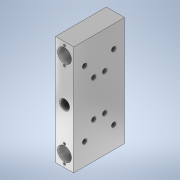
# Autodesk Inventor part: Bloque - Vinculo Cabezal
Saved by Autodesk Inventor 2020 (Build 240168000, 168)
## iProperties
Created: 2020-05-17
Part Number: Bloque - Vinculo Cabezal
Material: Aluminum 6061
Document SubType Name: Modeling
Designer: Dante
Density: 2.7 g/cm^3
Appearance: Aluminum - Dark
Mass: 559.283 g
Surface Area: 455.426 cm^2
Volume: 207.142 cm^3
Author: Dante
Autodesk Inventor part; units mm, degrees
ref_plane "YZ Plane" through (0, 0, 0) normal (1, 0, 0) x (0, 1, 0)
ref_plane "XZ Plane" through (0, 0, 0) normal (0, 1, 0) x (-1, 0, 0)
ref_plane "XY Plane" through (0, 0, 0) normal (0, 0, 1) x (1, 0, 0)
sketch "Sketch1" plane through (0, 0, 0) normal (0, 0, 1) x (1, 0, 0)
  line L0 (14.1854, 26.7901) -> (14.1854, -123.2099)
  line L1 (14.1854, -123.2099) -> (39.1854, -123.2099)
  line L2 (39.1854, -123.2099) -> (39.1854, 26.7901)
  line L3 (39.1854, 26.7901) -> (14.1854, 26.7901)
  circle A0 centre (26.6854, 10.2901) radius 9.5
  circle A1 centre (26.6854, -48.2099) radius 6
  circle A2 centre (37.1854, -8.2099) radius 3
  line L4 (39.1854, -5.2099) -> (14.1854, -5.2099)
  line L5 (39.1854, -11.2099) -> (14.1854, -11.2099)
  circle A3 centre (26.6854, 23.2901) radius 1.5
  line L6 (26.6854, 19.7901) -> (20.6854, 19.7901)
  line L7 (26.6854, 21.7901) -> (21.9472, 21.7901)
  line L8 (26.6854, 24.7901) -> (23.6854, 24.7901)
  line L9 (26.6854, 10.2901) -> (21.9472, 10.2901)
  circle A4 centre (26.6854, -2.7099) radius 1.5
  line L10 (14.1854, -48.2099) -> (17.1854, -48.2099)
  circle A5 centre (26.6854, -106.7099) radius 9.5
  circle A6 centre (37.1854, -88.2099) radius 3
  line L11 (39.1854, -91.2099) -> (14.1854, -91.2099)
  line L12 (39.1854, -85.2099) -> (14.1854, -85.2099)
  circle A7 centre (26.6854, -119.7099) radius 1.5
  line L13 (26.6854, -116.2099) -> (20.6854, -116.2099)
  line L14 (26.6854, -118.2099) -> (21.9472, -118.2099)
  line L15 (26.6854, -121.2099) -> (23.6854, -121.2099)
  line L16 (26.6854, -106.7099) -> (21.9472, -106.7099)
  circle A8 centre (26.6854, -93.7099) radius 1.5
  dimension "d0" = 150
  dimension "d1" = 25
  dimension "d6" = 12.5
  dimension "d8" = 12
  dimension "d12" = 75
  dimension "d13" = 6
  dimension "d33" = 3
  dimension "d81" = 3.5
  dimension "d83" = 2
  dimension "d84" = 2
  dimension "d85" = 16.5
  dimension "d130" = 12.5
  dimension "d131" = 12.5
  constraints: 34 end point, 16 symmetric about line, 8 horizontal, 7 centre point, 4 point on circle, 4 point on line, 3 perpendicular, 2 vertical alignment, 1 midpoint, 1 parallel, 1 tangent, 1 vertical, 8 other
  measures "d0" distance of L0.start L0.end
  measures "d1" distance of L0.end L1.end
  measures "d6" distance from line of L9.start L2
  measures "d8" diameter of A1
  measures "d12" distance from line of L3 A1.centre
  measures "d13" diameter of A2
  measures "d33" diameter of A3
  measures "d81" distance from line of L3 A3.centre
  measures "d83" distance between parallel lines of L3 L8
  measures "d84" distance between parallel lines of L6 L7
  measures "d85" distance from line of L3 L9.start
  measures "d130" distance from line of A1.centre L2
  measures "d131" distance from line of L16.start L2
extrude "Extrusion1" add sketch "Sketch1" along normal blind 70 contours L3 L2 L4 L0 | L4 A2 L5 L0 | L5 L2 L12 L0 | L4 L2 A2 | A2 L2 | A2 L2 L5 | L12 A6 L11 L0 | L11 L2 L1 L0 | L12 L2 A6 | A6 L2 | A6 L2 L11 | A3 | A4 | A7 | A8 picked at (35.982, -7.4645) picked at (36.2539, -87.8584)
sketch "Sketch2" plane through (39.1854, -123.2099, 0) normal (1, 0, 0) x (0, 0, -1)
  circle A0 centre (-27.5, 100) radius 3
  circle A1 centre (-42.5, 100) radius 3
  circle A2 centre (-55, 120) radius 3
  circle A3 centre (-15, 120) radius 3
  line L0 (0, 150) -> (-70, 150) projected
  line L1 (0, 0) -> (0, 150) projected
  line L2 (-70, 0) -> (-70, 150) projected
  line L3 (0, 75) -> (-12, 75)
  circle A4 centre (-27.5, 50) radius 3
  circle A5 centre (-42.5, 50) radius 3
  circle A6 centre (-55, 30) radius 3
  circle A7 centre (-15, 30) radius 3
  dimension "d17" = 6
  dimension "d18" = 6
  dimension "d19" = 6
  dimension "d20" = 6
  dimension "d21" = 30
  dimension "d24" = 30
  dimension "d25" = 15
  dimension "d26" = 15
  dimension "d204" = 50
  dimension "d205" = 50
  dimension "d206" = 12.5
  dimension "d207" = 12.5
  constraints: 8 centre point, 4 symmetric about line, 2 end point, 1 horizontal, 1 midpoint, 4 other
  measures "d17" diameter of A0
  measures "d18" diameter of A1
  measures "d19" diameter of A2
  measures "d20" diameter of A3
  measures "d21" distance from line of L0 A3.centre
  measures "d24" distance from line of L0 A2.centre
  measures "d25" distance from line of A3.centre L1
  measures "d26" distance from line of L2 A2.centre
  measures "d204" distance from line of L0 A1.centre
  measures "d205" distance from line of L0 A0.centre
  measures "d206" horizontal distance of A2.centre A1.centre
  measures "d207" horizontal distance of A3.centre A0.centre
sketch "Sketch5" plane through (0, 0, 0) normal (0, 0, -1) x (-1, 0, 0)
  circle A0 centre (-26.6854, 22.2901) radius 1.5
  line L0 (-39.1854, 26.7901) -> (-14.1854, 26.7901) projected
  circle A1 centre (-26.6854, 10.2901) radius 9.5 projected
  line L1 (-14.1854, 26.7901) -> (-14.1854, -123.2099) projected
  circle A2 centre (-26.6854, -1.7099) radius 1.5
  line L2 (-14.1854, 26.7901) -> (-14.1854, -123.2099) projected
  line L3 (-14.1854, -48.2099) -> (-19.6815, -48.2099)
  circle A3 centre (-26.6854, -118.7099) radius 1.5
  circle A4 centre (-26.6854, -94.7099) radius 1.5
  circle A5 centre (-26.6854, 10.2901) radius 9.5 projected
  line L4 (-26.6854, 0.7901) -> (-19.8619, 0.7901)
  dimension "d53" = 3
  dimension "d55" = 12.5
  dimension "d56" = 3
  dimension "d58" = 12.5
  dimension "d79" = 12
  dimension "d199" = 12
  constraints: 4 centre point, 4 end point, 3 horizontal, 2 symmetric about line, 1 midpoint, 1 vertical alignment, 3 other
  measures "d53" diameter of A0
  measures "d55" distance from line of A0.centre L1
  measures "d56" diameter of A2
  measures "d58" distance from line of A2.centre L1
  measures "d79" distance of A2.centre A1.centre
  measures "d199" distance of A1.centre A0.centre
sketch "Sketch7" plane through (0, 0, 70) normal (0, 0, 1) x (1, 0, 0)
  circle A0 centre (26.6854, 22.2901) radius 1.5
  line L0 (39.1854, 26.7901) -> (14.1854, 26.7901) projected
  line L1 (39.1854, -123.2099) -> (39.1854, 26.7901) projected
  circle A1 centre (26.6854, -1.7099) radius 1.5
  line L2 (39.1854, -48.2099) -> (34.5459, -48.2099)
  circle A2 centre (26.6854, -118.7099) radius 1.5
  line L3 (39.1854, -123.2099) -> (14.1854, -123.2099)
  line L4 (39.1854, 26.7901) -> (39.1854, -123.2099)
  line L5 (26.6854, -106.7099) -> (25.3096, -106.7099)
  circle A3 centre (26.6854, -94.7099) radius 1.5
  circle A4 centre (26.6854, 10.2901) radius 9.5 projected
  dimension "d87" = 3
  dimension "d89" = 12.5
  constraints: 8 end point, 5 symmetric about line, 4 centre point, 1 horizontal, 1 midpoint, 2 other
  measures "d87" diameter of A0
  measures "d89" distance from line of L1 A0.centre
thread "Thread16" size "M12x1.5" class "6H" standard "ISO Metric profile" length 40
sketch "Sketch8" plane through (0, 0, 0) normal (0, 0, -1) x (-1, 0, 0)
  line L0 (-39.1854, -48.2099) -> (-26.6854, -48.2099)
  circle A0 centre (-26.6854, -48.2099) radius 11
  circle A1 centre (-26.6854, -48.2099) radius 6 projected
  point P0 (0, 0)
  dimension "d113" = 12.5
  dimension "d114" = 22
  constraints: 2 end point, 1 centre point, 1 coincident, 1 concentric, 1 horizontal
  measures "d113" distance of L0.start L0.end
  measures "d114" diameter of A0
extrude "Extrusion9" cut sketch "Sketch8" against normal blind 10
sketch "Sketch9" plane through (0, 0, 0) normal (0, 0, -1) x (-1, 0, 0)
  circle A0 centre (-26.6854, -48.2099) radius 11
  circle A1 centre (-26.6854, -48.2099) radius 11 projected
  circle A2 centre (-26.6854, -34.2099) radius 1.5
  circle A3 centre (-26.6854, -62.2099) radius 1.5
  line L0 (-39.1854, -123.2099) -> (-39.1854, 26.7901) projected
  line L1 (-14.1854, 26.7901) -> (-14.1854, -123.2099) projected
  dimension "d117" = 22
  dimension "d118" = 3
  dimension "d119" = 3
  dimension "d120" = 14
  dimension "d121" = 14
  dimension "d122" = 12.5
  dimension "d123" = 12.5
  constraints: 3 centre point, 1 concentric
  measures "d117" diameter of A0
  measures "d118" diameter of A2
  measures "d119" diameter of A3
  measures "d120" distance of A2.centre A0.centre
  measures "d121" distance of A0.centre A3.centre
  measures "d122" distance from line of L0 A2.centre
  measures "d123" distance from line of L1 A3.centre
hole "Agujero1" at (39.1854, -3.2099, 55) at (39.1854, -23.2099, 42.5) at (39.1854, -23.2099, 27.5) at (39.1854, -3.2099, 15) at (39.1854, -93.2099, 55) at (39.1854, -73.2099, 42.5) at (39.1854, -73.2099, 27.5) at (39.1854, -93.2099, 15) direction (-1, 0, 0) diameter 6 depth 20 tip angle 118
hole "Agujero2" at (26.6854, -1.7099, 0) at (26.6854, 22.2901, 0) at (26.6854, -94.7099, 0) at (26.6854, -118.7099, 0) direction (0, 0, 1) diameter 3 depth 5 tip angle 118
thread "Rosca21" size "M3x0.5" class "6H" standard "ISO Metric profile" length 430
thread "Rosca22" size "M3x0.5" class "6H" standard "ISO Metric profile" length 430
thread "Rosca23" size "M3x0.5" class "6H" standard "ISO Metric profile" length 430
thread "Rosca24" size "M3x0.5" class "6H" standard "ISO Metric profile" length 430
hole "Agujero3" at (26.6854, 22.2901, 70) at (26.6854, -1.7099, 70) at (26.6854, -94.7099, 70) at (26.6854, -118.7099, 70) direction (0, 0, -1) diameter 3 depth 5 tip angle 118
thread "Rosca25" size "M3x0.5" class "6H" standard "ISO Metric profile" length 430
thread "Rosca26" size "M3x0.5" class "6H" standard "ISO Metric profile" length 430
thread "Rosca27" size "M3x0.5" class "6H" standard "ISO Metric profile" length 430
thread "Rosca28" size "M3x0.5" class "6H" standard "ISO Metric profile" length 430
hole "Agujero4" at (26.6854, -34.2099, 0) at (26.6854, -62.2099, 0) direction (0, 0, 1) diameter 3 depth 8 tip angle 118
thread "Rosca29" size "M3x0.5" class "6H" standard "ISO Metric profile" length 430
thread "Rosca30" size "M3x0.5" class "6H" standard "ISO Metric profile" length 430
sketch "Boceto10" plane through (0, 0, 70) normal (0, 0, 1) x (1, 0, 0)
  circle A0 centre (26.6854, -48.2099) radius 6 projected
  circle A1 centre (26.6854, -48.2099) radius 7
  point P0 (0, 0)
  dimension "d184" = 14
  constraints: 1 centre point, 1 coincident
  measures "d184" diameter of A1
hole "Agujero5" at (26.6854, -48.2099, 70) direction (0, 0, -1) diameter 14 depth 0.01 tip angle 118
sketch "Boceto11" plane through (14.1854, -123.2099, 0) normal (0, -1, 0) x (1, 0, 0)
  line L0 (6.5, 69.3891) -> (6.5, 10) projected
  circle A0 centre (3, 31) radius 1.5
  circle A1 centre (3, 39) radius 1.5
  line L1 (0, 0) -> (0, 70) projected
  line L2 (0, 70) -> (25, 70) projected
  point P0 (-14.1854, 0)
  dimension "d209" = 3
  dimension "d210" = 3
  dimension "d211" = 3
  dimension "d212" = 31
  dimension "d213" = 3
  dimension "d214" = 8
  constraints: 2 centre point
  measures "d209" diameter of A0
  measures "d210" diameter of A1
  measures "d211" distance from line of L1 A1.centre
  measures "d212" distance from line of L2 A1.centre
  measures "d213" distance from line of L1 A0.centre
  measures "d214" distance of A0.centre A1.centre
hole "Agujero7" at (17.1854, -123.2099, 31) at (17.1854, -123.2099, 39) direction (0, 1, 0) diameter 3 depth 10 tip angle 118
thread "Thread31" size "M3x0.5" class "6H" standard "ISO Metric profile" length 7
thread "Thread32" size "M3x0.5" class "6H" standard "ISO Metric profile" length 7
thread "Rosca33" size "M6x1" class "6H" standard "ANSI Metric M Profile" length 16
thread "Rosca34" size "M6x1" class "6H" standard "ANSI Metric M Profile" length 16
thread "Rosca35" size "M6x1" class "6H" standard "ANSI Metric M Profile" length 16
thread "Rosca36" size "M6x1" class "6H" standard "ANSI Metric M Profile" length 16
thread "Rosca37" size "M6x1" class "6H" standard "ANSI Metric M Profile" length 16
thread "Rosca38" size "M6x1" class "6H" standard "ANSI Metric M Profile" length 16
thread "Rosca39" size "M6x1" class "6H" standard "ANSI Metric M Profile" length 16
thread "Rosca40" size "M6x1" class "6H" standard "ANSI Metric M Profile" length 16
equation "\"d211\" = d213"
body "Solid1"
